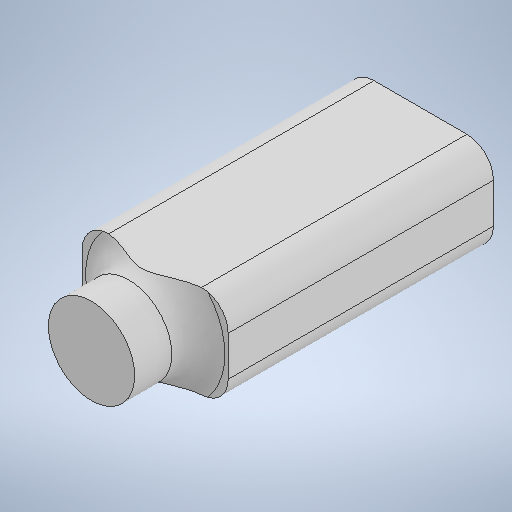
# Autodesk Inventor part: Cable_Usb_C
Saved by Autodesk Inventor 2025.2 (Build 292293000, 293)
## iProperties
Created: 2025-04-02
Part Number: Cable_Usb_C
Material: Generic
Document SubType Name: Modeling
Designer: ahorat
Density: 1 g/cm^3
Appearance: Default
Author: ahorat
Autodesk Inventor part; units mm, degrees
ref_plane "YZ Plane" through (0, 0, 0) normal (1, 0, 0) x (0, 1, 0)
ref_plane "XZ Plane" through (0, 0, 0) normal (0, 1, 0) x (-1, 0, 0)
ref_plane "XY Plane" through (0, 0, 0) normal (0, 0, 1) x (1, 0, 0)
sketch "Sketch1" plane through (0, 0, 0) normal (0, 0, 1) x (1, 0, 0)
  line L0 (-5.5, 3.5) -> (5.5, 3.5)
  line L1 (5.5, 3.5) -> (5.5, -3.5)
  line L2 (5.5, -3.5) -> (-5.5, -3.5)
  line L3 (-5.5, -3.5) -> (-5.5, 3.5)
  line L4 (-5.5, 3.5) -> (5.5, -3.5) construction
  line L5 (5.5, 3.5) -> (-5.5, -3.5) construction
  point P0 (0, 0)
  dimension "d0" = 11
  dimension "d1" = 7
  constraints: 12 end point, 2 midpoint, 2 parallel, 1 horizontal, 1 perpendicular
  measures "d0" distance of L0.start L0.end
  measures "d1" distance of L0.end L1.end
extrude "Extrusion1" add sketch "Sketch1" along normal blind 20
sketch "Sketch2" plane through (0, 0, 20) normal (0, 0, 1) x (1, 0, 0)
  circle A0 centre (0, 0) radius 3.25
  dimension "d4" = 6.5
  constraints: 1 centre point, 1 coincident
  measures "d4" diameter of A0
extrude "Extrusion2" add sketch "Sketch2" along normal blind 4.8
fillet "Fillet1" radius 2 5 edges at (5.5, 3.5, 10) (5.5, -3.5, 10) (-5.5, 3.5, 10) (-5.5, -3.5, 10) (-3.25, 0, 20)
body "Solid1"
